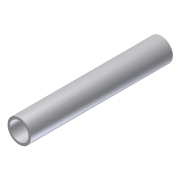
# Autodesk Inventor part: FE-00013-07
Saved by Autodesk Inventor 2012 (Build 160160000, 160)
## iProperties
Created: 2008-05-28
Part Number: FE-00013-07
Description: Coupling Extender
Document SubType Name: Modeling
Designer: narosenberg
Density: 1 g/cm^3
Mass: 65.7704 g
Surface Area: 391.083 cm^2
Volume: 65.7704 cm^3
Material: Default
Author: narosenberg
Autodesk Inventor part; units mm, degrees
ref_plane "XZ Plane" through (0, 0, 0) normal (0, 1, 0) x (-1, 0, 0)
ref_plane "XY Plane" through (0, 0, 0) normal (0, 0, 1) x (1, 0, 0)
sketch "Sketch1" plane through (0, 0, 0) normal (0, 0, 1) x (1, 0, 0)
  circle A0 centre (-14.7887, 6.8075) radius 16.764
  circle A1 centre (-14.7887, 6.8075) radius 13.335
  dimension "d0" = 33.528
  dimension "d1" = 26.67
  constraints: 2 centre point, 1 coincident
  measures "d0" diameter of A0
  measures "d1" diameter of A1
extrude "Extrusion1" add sketch "Sketch1" along normal blind 203.2
ref_plane "Work Plane1" through (-31.5527, 6.8075, 0) normal (1, 0, 0) x (0, 1, 0)
sketch "Sketch2" plane through (-31.5527, 6.8075, 0) normal (1, 0, 0) x (0, 1, 0)
  line L0 (16.764, 0) -> (16.764, 203.2) projected
  line L1 (-16.764, 203.2) -> (16.764, 203.2) projected
  line L2 (-16.764, 0) -> (16.764, 0) projected
  line L3 (0, 243.84) -> (0, -40.64) projected
  circle A0 centre (0, 88.9) radius 2.3813
  circle A1 centre (0, 114.3) radius 2.3813
  line L4 (16.764, 101.6) -> (-16.0957, 101.6)
  dimension "d4" = 101.6
  dimension "d5" = 12.7
  dimension "d6" = 12.7
  dimension "d7" = 4.7625
  dimension "d8" = 4.7625
  constraints: 2 centre point, 2 end point, 2 point on line, 1 midpoint, 1 perpendicular
  measures "d4" distance between parallel lines of L4 L1
  measures "d5" distance from line of A1.centre L4
  measures "d6" distance from line of A0.centre L4
  measures "d7" diameter of A0
  measures "d8" diameter of A1
extrude "Extrusion2" cut sketch "Sketch2" along normal up to next contours A0 L3 | L3 A0 | A1 L3 | L3 A1
body "Solid1"
